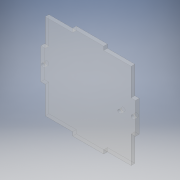
# Autodesk Inventor part: tapa superior
Saved by Autodesk Inventor 2016 (Build 200138000, 138)
## iProperties
Created: 2017-02-20
Part Number: tapa superior
Material: Generic
Document SubType Name: Modeling
Designer: jorge
Density: 1 g/cm^3
Appearance: Clear - Light
Author: jorge
## iProperties of the stored document tapa superior_3DPrint.ipt
Created: 2017-03-11
Part Number: tapa superior_3DPrint
Material: Generic
Document SubType Name: Modeling
Designer: jorge
Density: 1 g/cm^3
Appearance: Default
Author: jorge
Autodesk Inventor part; units mm, degrees
ref_plane "YZ Plane" through (0, 0, 0) normal (1, 0, 0) x (0, 1, 0)
ref_plane "XZ Plane" through (0, 0, 0) normal (0, 1, 0) x (-1, 0, 0)
ref_plane "XY Plane" through (0, 0, 0) normal (0, 0, 1) x (1, 0, 0)
sketch "Sketch1" plane through (0, 0, 0) normal (0, 0, 1) x (1, 0, 0)
  line L0 (0, 3) -> (25, 3) projected
  line L1 (0, 0) -> (0, 3) projected
  line L2 (25, 0) -> (25, 3) projected
  line L3 (25, 0) -> (47, 0) projected
  line L4 (47, 3) -> (47, -22) projected
  line L5 (47, -22) -> (50, -22) projected
  line L6 (50, -22) -> (50, -47) projected
  line L7 (47, -47) -> (50, -47) projected
  line L8 (47, -47) -> (47, -72) projected
  line L9 (25, -69) -> (47, -69) projected
  line L10 (25, -72) -> (25, -69) projected
  line L11 (0, -72) -> (25, -72) projected
  line L12 (0, -72) -> (0, -69) projected
  line L13 (-22, -69) -> (0, -69) projected
  line L14 (-22, -47) -> (-22, -72) projected
  line L15 (-25, -47) -> (-22, -47) projected
  line L16 (-25, -22) -> (-25, -47) projected
  line L17 (-25, -22) -> (-22, -22) projected
  line L18 (-22, 3) -> (-22, -22) projected
  line L19 (-22, 0) -> (0, 0) projected
  line L20 (-22, 0) -> (0, 0)
  line L21 (0, 0) -> (0, 3)
  line L22 (0, 3) -> (25, 3)
  line L23 (25, 3) -> (25, 0)
  line L24 (25, 0) -> (47, 0)
  line L25 (47, 0) -> (47, -22)
  line L26 (47, -22) -> (50, -22)
  line L27 (50, -47) -> (50, -22)
  line L28 (50, -47) -> (47, -47)
  line L29 (47, -47) -> (47, -69)
  line L30 (25, -69) -> (47, -69)
  line L31 (25, -69) -> (25, -72)
  line L32 (0, -72) -> (25, -72)
  line L33 (0, -72) -> (0, -69)
  line L34 (0, -69) -> (-22, -69)
  line L35 (-22, -47) -> (-25, -47)
  line L36 (-22, -47) -> (-22, -69)
  line L37 (-25, -47) -> (-25, -22)
  line L38 (-25, -22) -> (-22, -22)
  line L39 (-22, -22) -> (-22, 0)
  line L40 (0, 3) -> (0, 3)
  line L41 (0, 3) -> (0, 0)
  line L42 (25, 0) -> (25, 3)
  line L43 (25, 3) -> (25, 3)
  constraints: 48 end point, 14 perpendicular, 5 collinear, 2 horizontal, 2 vertical, 1 parallel
extrude "Extrusion1" add sketch "Sketch1" along normal blind 3
sketch "Sketch5" plane through (0, 0, 3) normal (0, 0, 1) x (1, 0, 0)
  line L0 (38.5, -12.7) -> (44.5, -12.7) projected
  line L1 (0, 0) -> (-22, 0) projected
  line L2 (-22, -47) -> (-22, -69) projected
  line L3 (47, -22) -> (47, 0) projected
  circle A0 centre (48.5, -34.5) radius 1.5
  circle A1 centre (12.5, -70.5) radius 1.5
  circle A2 centre (-23.5, -34.5) radius 1.5
  circle A3 centre (11, 1.5) radius 1.5
  line L4 (-22, 0) -> (-22, -22) projected
  line L5 (-22, -22) -> (-25, -22) projected
  line L6 (-25, -22) -> (-25, -47) projected
  line L7 (-25, -47) -> (-22, -47) projected
  line L8 (-22, -69) -> (0, -69) projected
  line L9 (0, -69) -> (0, -72) projected
  line L10 (0, -72) -> (25, -72) projected
  line L11 (25, -72) -> (25, -69) projected
  line L12 (25, -69) -> (47, -69) projected
  line L13 (47, -69) -> (47, -47) projected
  line L14 (47, -47) -> (50, -47) projected
  line L15 (50, -47) -> (50, -22) projected
  line L16 (50, -22) -> (47, -22) projected
  line L17 (47, 0) -> (25, 0) projected
  line L18 (25, 0) -> (25, 3) projected
  line L19 (25, 3) -> (0, 3) projected
  line L20 (0, 3) -> (0, 0) projected
  dimension "d12" = 3
  dimension "d13" = 3
  dimension "d14" = 3
  dimension "d15" = 3
  constraints: 4 centre point
  measures "d12" diameter of A0
  measures "d13" diameter of A1
  measures "d14" diameter of A2
  measures "d15" diameter of A3
extrude "Extrusion4" cut sketch "Sketch5" against normal blind 25.4 contours A2 | A0
sketch "Sketch6" plane through (0, 0, 3) normal (0, 0, 1) x (1, 0, 0)
  circle A0 centre (37.75, -35.9986) radius 1.5 projected
  point P0 (0, 0)
extrude "Extrusion5" cut sketch "Sketch6" against normal blind 3
sketch "Sketch7" plane through (50, -22, 3) normal (1, 0, 0) x (0, 0, -1)
  line L0 (3, -12.5) -> (3, 0) projected
  line L1 (0, -12.5) -> (3, -12.5) projected
  line L2 (3, -12.5) -> (3, 0) projected
  line L3 (3, 0) -> (0, 0) projected
  line L4 (0, -12.5) -> (0, 0) projected
  line L5 (0, -25) -> (0, -12.5) projected
  line L6 (3, -25) -> (0, -25) projected
  line L7 (3, -25) -> (3, -12.5) projected
  point P0 (3, 22)
extrude "Extrusion6" add sketch "Sketch7" along normal blind 0.5
sketch "Sketch8" plane through (-25, -22, 0) normal (-1, 0, 0) x (0, 0, 1)
  line L0 (3, -12.5) -> (0, -12.5) projected
  line L1 (3, 0) -> (3, -12.5) projected
  line L2 (0, 0) -> (3, 0) projected
  line L3 (0, 0) -> (0, -12.5) projected
  line L4 (0, -12.5) -> (0, -25) projected
  line L5 (0, -25) -> (3, -25) projected
  line L6 (3, -12.5) -> (3, -25) projected
  point P0 (0, 22)
extrude "Extrusion7" add sketch "Sketch8" along normal blind 0.5
body "Solid1"
